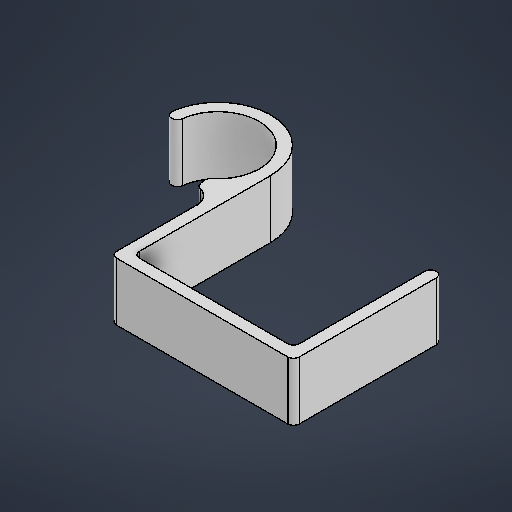
# Autodesk Inventor part: Clip
Saved by Autodesk Inventor 2026.1 (Build 301233000, 233)
## iProperties
Created: 2025-09-10
Part Number: Clip
Material: Generic
Document SubType Name: Modeling
Designer: JoshuaEah
Density: 1 g/cm^3
Appearance: Default
Author: JoshuaEah
Autodesk Inventor part; units mm, degrees
ref_plane "YZ Plane" through (0, 0, 0) normal (1, 0, 0) x (0, 1, 0)
ref_plane "XZ Plane" through (0, 0, 0) normal (0, 1, 0) x (-1, 0, 0)
ref_plane "XY Plane" through (0, 0, 0) normal (0, 0, 1) x (1, 0, 0)
sketch "Sketch1" plane through (0, 0, 0) normal (0, 1, 0) x (-1, 0, 0)
  circle A0 centre (0, 0) radius 18
  circle A1 centre (0, 0) radius 23
  line L0 (-98, 65) -> (-18, 65)
  line L1 (-18, 65) -> (-18, 0)
  line L2 (-98, 0) -> (-98, 65)
  line L3 (-23, 60) -> (-93, 60)
  line L4 (-93, 60) -> (-93, 0)
  line L5 (-23, 0) -> (-23, 60)
  line L6 (-93, 0) -> (-98, 0)
  line L7 (-18, 60) -> (-10.0531, 14.931)
  line L8 (23, 0) -> (-23, 0)
  point P0 (18, 0)
  point P1 (-10.9836, 20.2079)
  point P2 (-18, 14.3178)
  dimension "d0" = 36
  dimension "d1" = 5
  dimension "d10" = 5
  dimension "d11" = 5
  dimension "d13" = 60
  dimension "d14" = 70
  dimension "d15" = 10
  constraints: 18 end point, 4 perpendicular, 4 point on circle, 3 horizontal, 3 point on line, 2 centre point, 2 coincident, 2 tangent, 1 vertical
  measures "d0" diameter of A0
  measures "d1" radial gap between concentric circles of A1 A0
  measures "d10" distance between parallel lines of L0 L3
  measures "d11" distance between parallel lines of L2 L4
  measures "d13" distance of L5.start L3.start
  measures "d14" distance of L3.start L3.end
  measures "d15" angle of L1 L7
extrude "Extrusion1" add sketch "Sketch1" along normal mid plane 25.4 contours L8 A1 A0 | A0 L1 A1 L7 | L8 A1 L1 | A1 L5 L3 L4 L6 L2 L0 L1
fillet "Fillet1" radius 7.0104 1 edges at (18, 0, 14.3178)
extrude "Extrusion2" add sketch "Sketch1" along normal mid plane 3 contours A1 L1 L7
chamfer "Chamfer1" distance 3 angle 45 4 edges at (15.9446, 1.5, 22.2591) (18, 1.5, 43.6092) (15.9446, -1.5, 22.2591) (18, -1.5, 43.6092)
fillet "Fillet2" radius 2.5 11 edges at (18, 0, 65) (98, 0, 65) (98, 0, 0) (93, 0, 0) (23, 0, 60) (93, 0, 60) (-18, 0, 0) (-23, 0, 0) (10.0531, 0, 14.931) (10.9836, 8.6, 20.2079) (10.9836, -8.6, 20.2079)
equation "\"d10\" = d1"
equation "\"d11\" = d1"
body "Solid1"
